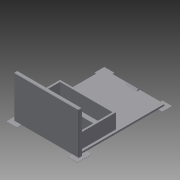
# Autodesk Inventor part: BOTTOM
Saved by Autodesk Inventor 2014 SP1 (Build 180222100, 222)
## iProperties
Created: 2013-12-02
Part Number: BOTTOM
Material: Generic
Document SubType Name: Modeling
Designer: Dominik
Density: 1 g/cm^3
Appearance: Default
Author: Dominik
Autodesk Inventor part; units mm, degrees
ref_plane "YZ Plane" through (0, 0, 0) normal (1, 0, 0) x (0, 1, 0)
ref_plane "XZ Plane" through (0, 0, 0) normal (0, 1, 0) x (-1, 0, 0)
ref_plane "XY Plane" through (0, 0, 0) normal (0, 0, 1) x (1, 0, 0)
sketch "Sketch1" plane through (0, 0, 0) normal (0, 0, 1) x (1, 0, 0)
  line L0 (0, 0) -> (55, 0)
  line L1 (55, 0) -> (55, 80)
  line L2 (55, 80) -> (0, 80)
  line L3 (0, 80) -> (0, 0)
  dimension "d0" = 55
  dimension "d1" = 80
  constraints: 8 end point
  measures "d0" distance between parallel lines of L1 L3
  measures "d1" distance between parallel lines of L0 L2
extrude "Base" add sketch "Sketch1" along normal blind 2
sketch "Sketch2" plane through (0, 0, 2) normal (0, 0, 1) x (1, 0, 0)
  line L0 (55, 0) -> (55, 80) projected
  line L1 (0, 80) -> (0, 0) projected
  line L2 (-2, 0) -> (57, 0)
  line L3 (57, 0) -> (57, 3)
  line L4 (57, 3) -> (-2, 3)
  line L5 (-2, 3) -> (-2, 0)
  dimension "d4" = 3
  dimension "d5" = 2
  dimension "d6" = 2
  constraints: 8 end point
  measures "d4" distance between parallel lines of L2 L4
  measures "d5" distance between parallel lines of L3 L0
  measures "d6" distance between parallel lines of L5 L1
extrude "Back" add sketch "Sketch2" along normal blind 36.5 and the other way blind 2
sketch "Sketch6" plane through (0, 0, 2) normal (0, 0, 1) x (1, 0, 0)
  line L0 (0, 80) -> (0, 3) projected
  line L1 (0, 3) -> (55, 3) projected
  line L2 (55, 3) -> (55, 80) projected
  line L3 (2, 3) -> (53, 3)
  line L4 (53, 3) -> (53, 38)
  line L5 (53, 38) -> (2, 38)
  line L6 (2, 38) -> (2, 3)
  point P0 (0, 0)
  dimension "d29" = 35
  dimension "d30" = 2
  dimension "d31" = 2
  constraints: 8 end point, 2 vertical, 1 horizontal, 1 point on line
  measures "d29" distance between parallel lines of L1 L5
  measures "d30" distance between parallel lines of L2 L4
  measures "d31" distance between parallel lines of L0 L6
extrude "Box" add sketch "Sketch6" along normal blind 13.5
chamfer "Chamfer3" distance 0.5 angle 45 8 edges at (0, 41.5, 0) (27.5, 80, 0) (55, 41.5, 0) (-1, 3, 0) (-2, 1.5, 0) (27.5, 0, 0) (57, 1.5, 0) (56, 3, 0)
chamfer "Chamfer4" distance 0.5 angle 45 3 edges at (-2, 0, 19.5) (27.5, 0, 38.5) (57, 0, 19.5)
chamfer "Chamfer5" distance 0.5 angle 45 3 edges at (-2, 1.75, 38.5) (27.5, 3, 38.5) (57, 1.75, 38.5)
sketch "Sketch7" plane through (0, 0, 15.5) normal (0, 0, 1) x (1, 0, 0)
  line L0 (53, 3) -> (2, 3) projected
  line L1 (53, 3) -> (53, 38) projected
  line L2 (53, 38) -> (2, 38) projected
  line L3 (2, 38) -> (2, 3) projected
  line L4 (3.6, 3) -> (51.4, 3)
  line L5 (51.4, 3) -> (51.4, 18.9)
  line L6 (51.4, 18.9) -> (3.6, 18.9)
  line L7 (3.6, 18.9) -> (3.6, 3)
  line L8 (51.4, 36.4) -> (3.6, 36.4)
  line L9 (3.6, 36.4) -> (3.6, 20.5)
  line L10 (3.6, 20.5) -> (51.4, 20.5)
  line L11 (51.4, 20.5) -> (51.4, 36.4)
  point P0 (0, 0)
  dimension "d44" = 1.6
  dimension "d45" = 1.6
  dimension "d46" = 1.6
  dimension "d47" = 1.6
  dimension "d48" = 1.6
  dimension "d49" = 1.6
  dimension "d50" = 15.9
  dimension "d51" = 15.9
  constraints: 16 end point, 1 point on line
  measures "d44" distance between parallel lines of L2 L8
  measures "d45" distance between parallel lines of L1 L11
  measures "d46" distance between parallel lines of L1 L5
  measures "d47" distance between parallel lines of L3 L7
  measures "d48" distance between parallel lines of L3 L9
  measures "d49" distance between parallel lines of L6 L10
  measures "d50" distance between parallel lines of L10 L8
  measures "d51" distance between parallel lines of L0 L6
extrude "Box inside" cut sketch "Sketch7" against normal blind 13.5 contours L0 L7 L6 L5 | L11 L10 L9 L8
sketch "Sketch8" plane through (0, 0, 2) normal (0, 0, 1) x (1, 0, 0)
  line L0 (55, 3) -> (55, 80) projected
  line L1 (55, 80) -> (0, 80) projected
  line L2 (0, 80) -> (0, 3) projected
  line L3 (22.5, 80) -> (32.5, 80)
  line L4 (32.5, 80) -> (32.5, 77.1)
  line L5 (32.5, 77.1) -> (22.5, 77.1)
  line L6 (22.5, 77.1) -> (22.5, 80)
  point P0 (0, 0)
  dimension "d63" = 22.5
  dimension "d64" = 22.5
  dimension "d65" = 10
  dimension "d66" = 2.9
  constraints: 8 end point, 1 point on line
  measures "d63" distance between parallel lines of L2 L6
  measures "d64" distance between parallel lines of L0 L4
  measures "d65" distance between parallel lines of L6 L4
  measures "d66" distance between parallel lines of L5 L1
extrude "Extrusion8" add sketch "Sketch8" along normal blind 1.5
chamfer "Chamfer9" distance 1.5 angle 45 1 edges at (27.5, 77.1, 3.5)
chamfer "Chamfer10" distance 1.4 angle 45 1 edges at (27.5, 80, 3.5)
sketch "Sketch9" plane through (0, 0, 0) normal (0, 0, -1) x (-1, 0, 0)
  line L0 (-58.372, 83.6354) -> (-49.5119, 83.6354)
  line L1 (-49.5119, 83.6354) -> (-49.5119, 74.6368)
  line L2 (-49.5119, 74.6368) -> (-58.372, 74.6368)
  line L3 (-58.372, 74.6368) -> (-58.372, 83.6354)
  line L4 (-5.9034, 83.6354) -> (3.372, 83.6354)
  line L5 (3.372, 83.6354) -> (3.372, 74.6368)
  line L6 (3.372, 74.6368) -> (-5.9034, 74.6368)
  line L7 (-5.9034, 74.6368) -> (-5.9034, 83.6354)
  line L8 (-4.6575, 9.1548) -> (5.0333, 9.1548)
  line L9 (5.0333, 9.1548) -> (5.0333, -3.8585)
  line L10 (5.0333, -3.8585) -> (-4.6575, -3.8585)
  line L11 (-4.6575, -3.8585) -> (-4.6575, 9.1548)
  line L12 (-50.8963, 9.1548) -> (-59.7564, 9.1548)
  line L13 (-59.7564, 9.1548) -> (-59.7564, -3.8585)
  line L14 (-59.7564, -3.8585) -> (-50.8963, -3.8585)
  line L15 (-50.8963, -3.8585) -> (-50.8963, 9.1548)
  point P0 (0, 0)
  constraints: 32 end point
extrude "printing support" add sketch "Sketch9" against normal blind 0.2
equation "\"d31\" = d30"
equation "\"d45\" = d44"
equation "\"d46\" = d45"
equation "\"d47\" = d46"
equation "\"d48\" = d44"
equation "\"d49\" = d44"
equation "\"d64\" = d63"
body "Solid1"
